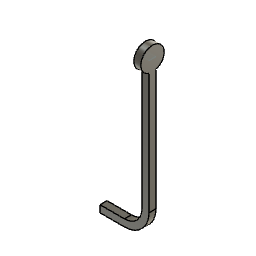
back link v3 (Autodesk Fusion 360 design; units mm, degrees)
Autodesk Fusion 360 part; units mm, degrees
sketch "Sketch1" plane through (0, 0, 0) normal (1, 0, 0) x (0, 1, 0)
  line L0 (7.5, -7.5) -> (-7.5, -7.5)
  line L1 (-7.5, -7.5) -> (-7.5, 7.5)
  line L2 (-7.5, 7.5) -> (7.5, 7.5)
  line L3 (7.5, 7.5) -> (7.5, -7.5)
  line L4 (7.5, -7.5) -> (-7.5, 7.5) construction
  line L5 (-7.5, -7.5) -> (7.5, 7.5) construction
  dimension "d1" = 15
  dimension "d2" = 15
  constraint horizontal L0
  constraint perpendicular L0 L1
  constraint parallel L0 L2
  constraint parallel L1 L3
  constraint coincident L4 origin
  constraint coincident L5 origin
  measures "d1" distance of L1.end L2.end
  measures "d2" distance of L0.end L1.end
sketch "Sketch2" plane through (0, 0, 0) normal (0, 1, 0) x (1, 0, 0)
  line L0 (0, -7.5) -> (52.5, -7.5)
  line L1 (90, -45) -> (90, -257.5)
  arc A0 (90, -45) -> (52.5, -7.5) centre (52.5, -45) ccw
  point P0 (90, -7.5)
  dimension "d3" = 7.5
  dimension "d4" = 90
  dimension "d5" = 250
  dimension "d6" = 37.5
  constraint perpendicular L0 L1
  constraint coincident P0 L1
  constraint coincident P0 L0
  constraint tangent L1 A0
  constraint tangent L0 A0
  measures "d3" distance of origin L0.start
  measures "d4" distance of L0.start P0
  measures "d5" distance of P0 L1.end
  measures "d6" radius of A0
sweep "Sweep1" add profiles "Sketch1" path "Sketch2" along L1 A0 L0 section 1
extrude "Extrude1" add 1 faces at (95, 2.5, 257.5) along direction (0, 0, 1) blind 50
extrude "Extrude2" add 1 faces at (95, 2.5, 307.5) along direction (0, 0, 1) blind 20
ref_plane "WorkPlane1" through (90, 7.5, 327.5) normal (1, 0, 0) x (0, 1, 0)
sketch "Sketch4" plane through (0, 0, 327.5) normal (0, 0, 1) x (-1, 0, 0)
  line L0 (-90, -7.5) -> (-90, 7.5)
  line L1 (-90, 7.5) -> (-105, 7.5)
  line L2 (-105, 7.5) -> (-105, -7.5)
  line L3 (-105, -7.5) -> (-90, -7.5)
sketch "Sketch3" plane through (90, 7.5, 327.5) normal (1, 0, 0) x (0, 1, 0)
  circle A0 centre (-7.5, 0) radius 25
  point P0 (-7.5, 0)
  dimension "d17" = 50
  constraint coincident P0 A0.centre
  measures "d17" diameter of A0
extrude "Extrude3" add sketch "Sketch3" along normal blind 15
